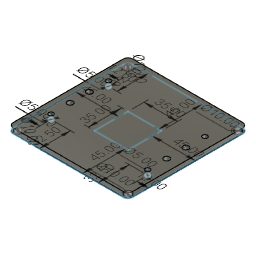
Main_plate (Autodesk Fusion 360 design; units mm, degrees)
Autodesk Fusion 360 part; units mm, degrees
sketch "Sketch1" plane through (0, 0, 0) normal (0, 0, 1) x (1, 0, 0)
  line L0 (5, 0) -> (120, 0)
  line L1 (125, 5) -> (125, 120)
  line L2 (120, 125) -> (5, 125)
  line L3 (0, 120) -> (0, 5)
  arc A0 (125, 120) -> (120, 125) centre (120, 120) ccw
  arc A1 (5, 125) -> (0, 120) centre (5, 120) ccw
  arc A2 (0, 5) -> (5, 0) centre (5, 5) ccw
  arc A3 (120, 0) -> (125, 5) centre (120, 5) ccw
  circle A4 centre (12, 32.5) radius 2.5
  circle A5 centre (113, 32.5) radius 2.5
  circle A6 centre (12, 92.5) radius 2.5
  line L4 (45, 80) -> (80, 80)
  line L5 (80, 80) -> (80, 45)
  line L6 (80, 45) -> (45, 45)
  line L7 (45, 45) -> (45, 80)
  dimension "d3" = 10
  dimension "d4" = 10
  dimension "d5" = 10
  dimension "d6" = 10
  dimension "d7" = 5
  dimension "d8" = 12
  dimension "d9" = 32.5
  dimension "d10" = 5
  dimension "d11" = 12
  dimension "d12" = 32.5
  dimension "d13" = 5
  dimension "d15" = 12
  dimension "d16" = 32.5
  dimension "d81" = 35
  dimension "d82" = 35
  dimension "d83" = 45
  dimension "d84" = 45
  dimension "d85" = 45
  dimension "d86" = 45
  constraint horizontal L0
  constraint vertical L1
  constraint horizontal L2
  constraint vertical L3
  constraint tangent L2 A0
  constraint tangent L1 A0
  constraint tangent L2 A1
  constraint tangent L3 A1
  constraint tangent L3 A2
  constraint tangent L0 A2
  constraint tangent L1 A3
  constraint tangent L0 A3
  constraint horizontal L4
  constraint vertical L5
  constraint horizontal L6
  constraint vertical L7
  measures "d3" diameter of A0
  measures "d4" diameter of A1
  measures "d5" diameter of A2
  measures "d6" diameter of A3
  measures "d7" diameter of A4
  measures "d8" distance of L3 A4.centre
  measures "d9" distance of L0 A4.centre
  measures "d10" diameter of A5
  measures "d11" distance of L1 A5.centre
  measures "d12" distance of L0 A5.centre
  measures "d13" diameter of A6
  measures "d15" distance of L3 A6.centre
  measures "d16" distance of L2 A6.centre
  measures "d81" distance of L4.start L4.end
  measures "d82" distance of L4.start L6.end
  measures "d83" distance of L0 L6
  measures "d84" distance of L3 L7
  measures "d85" distance of L1 L5
  measures "d86" distance of L2 L4
extrude "Extrude1" add sketch "Sketch1" along normal blind 5 contours L0 L1 L2 L3 A0 A1 A2 A3 | L4 L5 L6 L7
sketch "Sketch2" plane through (0, 0, 5) normal (0, 0, 1) x (-1, 0, 0)
  circle A0 centre (-12, -72.5) radius 3
  line L0 (0, -120) -> (0, -5)
  circle A1 centre (-12, -52.5) radius 3
  circle A2 centre (-113, -52.5) radius 3
  line L1 (-125, -5) -> (-125, -120)
  circle A3 centre (-113, -72.5) radius 3
  circle A4 centre (-113, -92.5) radius 2.5
  line L2 (-120, -125) -> (-5, -125)
  point P0 (-12, -92.5)
  point P1 (-12, -32.5)
  point P2 (-113, -32.5)
  dimension "d65" = 6
  dimension "d66" = 20
  dimension "d67" = 12
  dimension "d68" = 6
  dimension "d69" = 20
  dimension "d70" = 12
  dimension "d71" = 20
  dimension "d72" = 6
  dimension "d73" = 12
  dimension "d74" = 6
  dimension "d75" = 12
  dimension "d148" = 5
  dimension "d149" = 20
  dimension "d150" = 20
  dimension "d151" = 20
  dimension "d152" = 32.5
  dimension "d153" = 12
  measures "d65" diameter of A0
  measures "d66" vertical distance of A0.centre P0
  measures "d67" distance of A0.centre L0
  measures "d68" diameter of A1
  measures "d69" vertical distance of A0.centre A1.centre
  measures "d70" distance of L0 A1.centre
  measures "d71" distance of A1.centre P1
  measures "d72" diameter of A2
  measures "d73" distance of A2.centre L1
  measures "d74" diameter of A3
  measures "d75" distance of L1 A3.centre
  measures "d148" diameter of A4
  measures "d149" vertical distance of A3.centre A4.centre
  measures "d150" distance of A2.centre A3.centre
  measures "d151" vertical distance of A2.centre P2
  measures "d152" distance of A4.centre L2
  measures "d153" distance of L1 A4.centre
sketch "Sketch3" plane through (0, 0, 5) normal (0, 0, 1) x (-1, 0, 0)
extrude "Extrude2" add sketch "Sketch2" against normal blind 5 contours A0 | A1 | A2 | A3
extrude "Extrude3" cut sketch "Sketch2" against normal blind 5 contours A0 | A1 | A2 | A3
sketch "Sketch4" plane through (0, 0, 5) normal (0, 0, 1) x (-1, 0, 0)
  circle A0 centre (-113, -92.5) radius 2.5
  line L0 (-120, -125) -> (-5, -125)
  line L1 (-125, -5) -> (-125, -120)
  dimension "d145" = 5
  dimension "d146" = 32.5
  dimension "d147" = 12
  measures "d145" diameter of A0
  measures "d146" distance of A0.centre L0
  measures "d147" distance of A0.centre L1
extrude "Extrude4" cut sketch "Sketch4" against normal blind 5
equation "main_plate_thickness = 5 mm"
equation "d77 = -main_plate_thickness"
equation "d79 = -main_plate_thickness"
